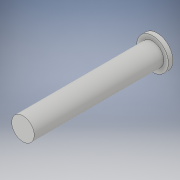
# Autodesk Inventor part: axle_TX2437
Saved by Autodesk Inventor 2018 (Build 220112000, 112)
## iProperties
Created: 2018-03-22
Part Number: axle_TX2437
Material: Generic
Document SubType Name: Modeling
Designer: dvyen
Density: 1 g/cm^3
Appearance: Default
Author: dvyen
Autodesk Inventor part; units mm, degrees
ref_plane "YZ Plane" through (0, 0, 0) normal (1, 0, 0) x (0, 1, 0)
ref_plane "XZ Plane" through (0, 0, 0) normal (0, 1, 0) x (-1, 0, 0)
ref_plane "XY Plane" through (0, 0, 0) normal (0, 0, 1) x (1, 0, 0)
sketch "Sketch1" plane through (0, 0, 0) normal (0, 0, 1) x (1, 0, 0)
  circle A0 centre (0, 0) radius 2.49
  circle A1 centre (0, 0) radius 3.5
  dimension "d0" = 4.98
  dimension "d1" = 7
  constraints: 2 centre point, 2 coincident
  measures "d0" diameter of A0
  measures "d1" diameter of A1
extrude "Extrusion1" add sketch "Sketch1" along normal blind 1
sketch "Sketch2" plane through (0, 0, 0) normal (0, 0, 1) x (1, 0, 0)
  circle A0 centre (0, 0) radius 2.49
  constraints: 1 centre point, 1 coincident
extrude "Extrusion2" add sketch "Sketch2" along normal blind 29.6
body "Solid1"
